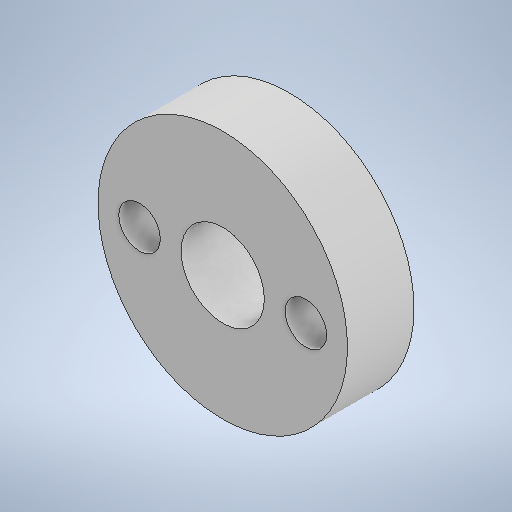
# Autodesk Inventor part: set_10_28
Saved by Autodesk Inventor 2025.1 (Build 291241000, 241)
## iProperties
Created: 2025-05-06
Part Number: set_10_28
Material: 一般
Document SubType Name: Modeling
Designer: yuki0520
Density: 1 g/cm^3
Appearance: 既定
Author: yuki0520
Autodesk Inventor part; units mm, degrees
ref_plane "YZ Plane" through (0, 0, 0) normal (1, 0, 0) x (0, 1, 0)
ref_plane "XZ Plane" through (0, 0, 0) normal (0, 1, 0) x (-1, 0, 0)
ref_plane "XY Plane" through (0, 0, 0) normal (0, 0, 1) x (1, 0, 0)
sketch "スケッチ1" plane through (0, 0, 0) normal (0, 0, 1) x (1, 0, 0)
  circle A0 centre (0, 0) radius 5
  circle A1 centre (0, 0) radius 15
  circle A2 centre (0, 0) radius 10
  circle A3 centre (10, 0) radius 2.5
  circle A4 centre (-10, 0) radius 2.5
  line L0 (-10, 0) -> (10, 0)
  dimension "d0" = 10
  dimension "d1" = 30
  dimension "d2" = 20
  dimension "d3" = 5
  dimension "d4" = 5
  constraints: 5 centre point, 3 coincident, 3 point on circle, 2 end point, 1 horizontal, 1 midpoint, 1 point on line
  measures "d0" diameter of A0
  measures "d1" diameter of A1
  measures "d2" diameter of A2
  measures "d3" diameter of A3
  measures "d4" diameter of A4
extrude "押し出し1" add sketch "スケッチ1" along normal blind 8 contours L0 A3 A2 A4 A0 | A0 L0 A4 A2 A3 | A1
